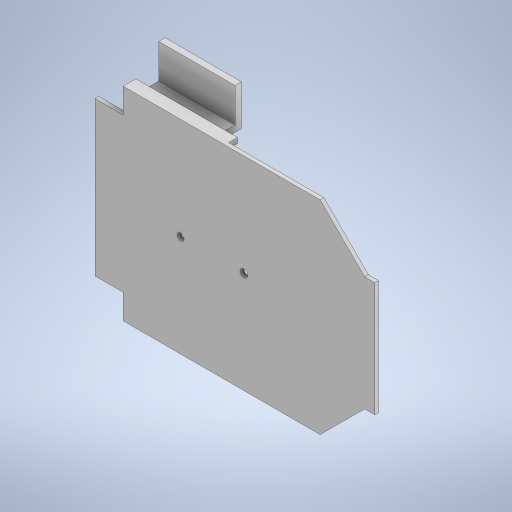
# Autodesk Inventor part: boschprofil-platform
Saved by Autodesk Inventor 2024 (Build 280153000, 153)
## iProperties
Created: 2024-04-17
Part Number: boschprofil-platform
Material: Generisch
Document SubType Name: Modeling
Designer: anash
Density: 1 g/cm^3
Appearance: Vorgabe
Author: anash
Autodesk Inventor part; units mm, degrees
ref_plane "YZ Plane" through (0, 0, 0) normal (1, 0, 0) x (0, 1, 0)
ref_plane "XZ Plane" through (0, 0, 0) normal (0, 1, 0) x (-1, 0, 0)
ref_plane "XY Plane" through (0, 0, 0) normal (0, 0, 1) x (1, 0, 0)
sketch "Skizze1" plane through (0, 0, 0) normal (0, 1, 0) x (-1, 0, 0)
  circle A0 centre (-117, -80) radius 3
  circle A1 centre (-67.25, -80) radius 2.75
  line L0 (-170, -160) -> (-22, -160)
  line L1 (-220, -125) -> (-212, -125)
  line L2 (-212, -35) -> (-220, -35)
  line L3 (-220, -35) -> (-220, -125)
  line L4 (0, -19.5) -> (-22, -19.5)
  line L5 (-212, -35) -> (-177, 0)
  line L6 (-212, -125) -> (-177, -160)
  line L7 (-22, -140.5) -> (0, -140.5)
  line L8 (-22, 0) -> (-22, -15.5)
  line L9 (-22, -19.5) -> (0, -19.5)
  line L10 (-22, -160) -> (-22, -144.5)
  line L11 (-22, -140.5) -> (0, -140.5)
  line L12 (-22, 0) -> (-102, 0)
  line L13 (-102, 0) -> (-102, -4)
  line L14 (-22, -15.5) -> (-22, 0)
  line L15 (-22, -160) -> (-102, -160)
  line L16 (-102, -160) -> (-102, -156)
  line L17 (-22, -144.5) -> (-22, -160)
  line L18 (-22, -160) -> (-102, -160)
  line L19 (-102, -160) -> (-102, -156)
  line L20 (-102, -156) -> (-22, -156)
  line L21 (-22, -156) -> (-22, -160)
  line L22 (-22, -156) -> (-102, -156)
  line L23 (-22, -149.5) -> (-22, -156)
  line L24 (-22, 0) -> (-102, 0)
  line L25 (-102, 0) -> (-102, -4)
  line L26 (-102, -4) -> (-22, -4)
  line L27 (-22, -4) -> (-22, 0)
  line L28 (-22, -4) -> (-102, -4)
  line L29 (-22, -10.5) -> (-22, -4)
  line L30 (-22, -15.5) -> (-22, -10.5)
  line L31 (-22, -149.5) -> (-82, -149.5)
  line L32 (-22, -144.5) -> (-22, -149.5)
  line L33 (-22, -144.5) -> (-22, -140.5)
  line L34 (-22, 0) -> (-177, 0)
  line L35 (-22, 0) -> (-170, 0)
  line L36 (-22, -15.5) -> (-22, -19.5)
  line L37 (0, -19.5) -> (0, -140.5)
  line L38 (-22, -144.5) -> (-82, -144.5)
  line L39 (-82, -144.5) -> (-82, -149.5)
  line L40 (-82, -149.5) -> (-22, -149.5)
  line L41 (-22, -149.5) -> (-22, -144.5)
  line L42 (-22, -15.5) -> (-82, -15.5)
  line L43 (-82, -15.5) -> (-82, -10.5)
  line L44 (-82, -10.5) -> (-22, -10.5)
  line L45 (-22, -10.5) -> (-22, -15.5)
  line L46 (-82, -15.5) -> (-22, -15.5)
  line L47 (-82, -144.5) -> (-22, -144.5)
  line L48 (-82, -10.5) -> (-22, -10.5)
  line L49 (-220, -35) -> (-220, -125)
  line L50 (-177, -160) -> (-22, -160)
  point P0 (0, 0)
  point P1 (-216, -125)
  point P2 (-216, -35)
  point P3 (-22, -4)
  dimension "d4" = 6
  dimension "d5" = 49.75
  dimension "d7" = 5.5
  dimension "d9" = 8
  dimension "d10" = 90
  dimension "d14" = 60.5
  dimension "d15" = 60.5
  dimension "d17" = 35
  dimension "d25" = 4
  dimension "d27" = 4
  dimension "d31" = 60
  dimension "d32" = 60
  constraints: 102 end point, 16 parallel, 13 horizontal, 8 perpendicular, 3 point on line, 2 centre point, 2 midpoint, 1 collinear, 1 vertical
  measures "d4" diameter of A0
  measures "d5" distance of A0.centre A1.centre
  measures "d7" diameter of A1
  measures "d9" distance of L2.end L2.start
  measures "d10" distance of L2.start L1.end
  measures "d14" distance from line of L4 A1.centre
  measures "d15" distance from line of L4 A0.centre
  measures "d17" horizontal distance of L2.start L5.end
  measures "d25" distance of L18.end L19.end
  measures "d27" distance of L25.end L24.end
  measures "d31" distance of L40.end L31.end
  measures "d32" distance of L43.end L44.end
extrude "Extrusion1" add sketch "Skizze1" along normal blind 3 contours L50 L6 L1 L3 L2 L5 L34 L13 L26 L8 L44 L43 L42 L36 L4 L37 L7 L33 L38 L39 L31 L10 L20 L16 L0
sketch "Skizze2" plane through (0, 0, 0) normal (0, -1, 0) x (1, 0, 0)
  line L0 (22, -15.5) -> (82, -15.5) projected
  line L1 (82, -15.5) -> (82, -10.5) projected
  line L2 (22, -15.5) -> (82, -15.5)
  line L3 (82, -15.5) -> (82, -10.5)
  line L4 (82, -10.5) -> (22, -10.5)
  line L5 (22, -10.5) -> (22, -15.5)
  line L6 (22, -149.5) -> (82, -149.5) projected
  line L7 (82, -144.5) -> (22, -144.5) projected
  line L8 (22, -149.5) -> (82, -149.5)
  line L9 (82, -149.5) -> (82, -144.5)
  line L10 (82, -144.5) -> (22, -144.5)
  line L11 (22, -144.5) -> (22, -149.5)
  line L12 (102, -156) -> (22, -156) projected
  line L13 (177, -160) -> (102, -160) projected
  line L14 (22, -156) -> (102, -156)
  line L15 (102, -156) -> (102, -160)
  line L16 (102, -160) -> (22, -160)
  line L17 (22, -160) -> (22, -156)
  line L18 (22, -4) -> (102, -4) projected
  line L19 (102, 0) -> (177, 0) projected
  line L20 (22, -4) -> (102, -4)
  line L21 (102, -4) -> (102, 0)
  line L22 (102, 0) -> (22, 0)
  line L23 (22, 0) -> (22, -4)
  point P0 (0, 0)
  constraints: 32 end point, 8 parallel, 4 horizontal, 4 perpendicular
extrude "Extrusion2" add sketch "Skizze2" against normal blind 10 contours L15 L16 L17 L12 | L23 L22 L21 L18
sketch "Skizze3" plane through (0, 0, 0) normal (0, -1, 0) x (1, 0, 0)
  line L0 (82, -15.5) -> (82, -10.5) projected
  line L1 (22, -15.5) -> (82, -15.5)
  line L2 (82, -15.5) -> (82, -10.5)
  line L3 (82, -10.5) -> (22, -10.5)
  line L4 (22, -10.5) -> (22, -15.5)
  line L5 (82, -144.5) -> (22, -144.5) projected
  line L6 (82, -149.5) -> (82, -144.5) projected
  line L7 (22, -144.5) -> (82, -144.5)
  line L8 (82, -144.5) -> (82, -149.5)
  line L9 (82, -149.5) -> (22, -149.5)
  line L10 (22, -149.5) -> (22, -144.5)
  point P0 (0, 0)
  constraints: 16 end point, 4 parallel, 2 horizontal, 2 perpendicular
extrude "Extrusion3" add sketch "Skizze3" against normal blind 33
sketch "Skizze4" plane through (22, 3, -10.5) normal (0, 0, 1) x (1, 0, 0)
  line L0 (0, 0) -> (0, 30) projected
  line L1 (60, 0) -> (60, 30) projected
  line L2 (0, 30) -> (60, 30)
  line L3 (60, 30) -> (60, 25)
  line L4 (60, 25) -> (0, 25)
  line L5 (0, 25) -> (0, 30)
  point P0 (-22, -3)
  dimension "d39" = 5
  constraints: 8 end point, 2 parallel, 1 horizontal, 1 perpendicular, 1 point on line
  measures "d39" distance of L2.end L3.end
extrude "Extrusion4" add sketch "Skizze4" along normal blind 27
sketch "Skizze5" plane through (82, 3, -149.5) normal (0, 0, -1) x (-1, 0, 0)
  line L0 (0, 0) -> (0, 30) projected
  line L1 (60, 0) -> (60, 30) projected
  line L2 (0, 30) -> (60, 30)
  line L3 (60, 30) -> (60, 25)
  line L4 (60, 25) -> (0, 25)
  line L5 (0, 25) -> (0, 30)
  point P0 (82, -3)
  dimension "d42" = 5
  constraints: 8 end point, 2 parallel, 1 horizontal, 1 perpendicular, 1 point on line
  measures "d42" distance of L2.end L3.end
extrude "Extrusion5" add sketch "Skizze5" along normal blind 27
